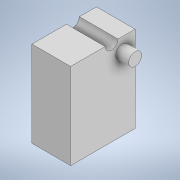
# Autodesk Inventor part: Support_1A
Saved by Autodesk Inventor 2021 (Build 250183000, 183)
## iProperties
Created: 2021-04-14
Part Number: Support_1A
Material: Generic
Document SubType Name: Modeling
Designer: Jawal
Density: 1 g/cm^3
Appearance: Default
Author: Jawal
Autodesk Inventor part; units mm, degrees
note: some values were not read from the file. Chosen so that the rebuilt part matches the saved one: direction of "Emboss1".
ref_plane "YZ Plane" through (0, 0, 0) normal (1, 0, 0) x (0, 1, 0)
ref_plane "XZ Plane" through (0, 0, 0) normal (0, 1, 0) x (-1, 0, 0)
ref_plane "XY Plane" through (0, 0, 0) normal (0, 0, 1) x (1, 0, 0)
sketch "Sketch1" plane through (0, 0, 0) normal (1, 0, 0) x (0, 1, 0)
  line L0 (10.5655, 7.5) -> (-10.5655, 7.5)
  line L1 (-10.5655, 7.5) -> (-10.5655, -6.983)
  line L2 (-10.5655, -6.983) -> (10.5655, -6.983)
  line L3 (10.5655, -6.983) -> (10.5655, 7.5)
  point P0 (0, 0)
  dimension "d0" = 21.131
  dimension "d2" = 10.5655
  dimension "d3" = 7.5
  dimension "d27" = 14.483
  constraints: 8 end point, 2 parallel, 1 horizontal, 1 perpendicular
  measures "d0" distance of L1.end L2.end
  measures "d2" distance from line of L3 point (0, 0)
  measures "d3" distance from line of L0 point (0, 0)
  measures "d27" distance of L0.start L2.end
extrude "Extrusion1" add sketch "Sketch1" along normal blind 9
sketch "Sketch3" plane through (9, 0, 0) normal (1, 0, 0) x (0, 0, -1)
  circle A0 centre (3.983, 6.2605) radius 1.5
  point P0 (0, 0)
  dimension "d12" = 3
  constraints: 1 centre point
  measures "d12" diameter of A0
extrude "Extrusion3" add sketch "Sketch3" along normal blind 3
sketch "Sketch4" plane through (0, 0, 0) normal (-1, 0, 0) x (0, 0, 1)
  line L0 (-2.5186, -3.6831) -> (10.3419, -3.6831) construction
  line L1 (10.3419, -3.6831) -> (10.3419, -8.8157) construction
  line L2 (10.3419, -8.8157) -> (-2.5186, -8.8157) construction
  line L3 (-2.5186, -8.8157) -> (-2.5186, -3.6831) construction
  line L4 (-0.5697, -6.741) -> (-2.0567, -6.741)
  line L5 (-2.0567, -6.741) -> (-2.0567, -6.4297)
  line L6 (-2.0567, -6.4297) -> (-1.5034, -6.4297)
  line L7 (-1.5034, -6.4297) -> (-1.5034, -4.387)
  line L8 (-1.5034, -4.387) -> (-2.0567, -4.387)
  line L9 (-2.0567, -4.387) -> (-2.0567, -4.1079)
  spline S0 degree 2 poles (-2.0567, -4.1079) (-1.743, -4.1079) (-1.4466, -3.9301) (-1.4268, -3.6831) knots 0 0 0 1 2 2 2
  line L10 (-1.4268, -3.6831) -> (-1.1106, -3.6831)
  line L11 (-1.1106, -3.6831) -> (-1.1106, -6.4297)
  line L12 (-1.1106, -6.4297) -> (-0.5697, -6.4297)
  line L13 (-0.5697, -6.4297) -> (-0.5697, -6.741)
  line L14 (-0.2511, -6.741) -> (0.7764, -3.693)
  line L15 (0.7764, -3.693) -> (1.2754, -3.693)
  line L16 (1.2754, -3.693) -> (2.3029, -6.741)
  line L17 (2.3029, -6.741) -> (1.8756, -6.741)
  line L18 (1.8756, -6.741) -> (1.599, -5.8888)
  line L19 (1.599, -5.8888) -> (0.4356, -5.8888)
  line L20 (0.4356, -5.8888) -> (0.1589, -6.741)
  line L21 (0.1589, -6.741) -> (-0.2511, -6.741)
  line L22 (1.4878, -5.543) -> (1.016, -4.1079)
  line L23 (1.016, -4.1079) -> (0.5467, -5.543)
  line L24 (0.5467, -5.543) -> (1.4878, -5.543)
  point P0 (0, 0)
  constraints: 2 other
emboss "Emboss1" sketch "Sketch4" operation cut depth 1 direction (1, 0, 0)
sketch "Sketch6" plane through (0, -10.5655, -6.983) normal (0, -1, 0) x (1, 0, 0)
  line L0 (0, 14.483) -> (0, 0) projected
  line L1 (9, 14.483) -> (9, 0) projected
  line L2 (0, 0) -> (9, 0)
  line L3 (9, 0) -> (9, 14.483)
  line L4 (9, 14.483) -> (0, 14.483)
  line L5 (0, 14.483) -> (0, 0)
  point P0 (0, 6.983)
  constraints: 8 end point, 2 parallel, 1 horizontal, 1 perpendicular
extrude "Extrusion5" add sketch "Sketch6" along normal blind 0.174
sketch "Sketch7" plane through (0, 10.5655, 7.5) normal (0, 0, 1) x (1, 0, 0)
  line L0 (0, 0) -> (9, 0) projected
  line L1 (9, 0) -> (9, -21.305) projected
  line L2 (0, 0) -> (9, 0)
  line L3 (9, 0) -> (9, -21.305)
  line L4 (9, -21.305) -> (0, -21.305)
  line L5 (0, -21.305) -> (0, 0)
  point P0 (0, -10.5655)
  constraints: 8 end point, 2 parallel, 1 horizontal, 1 perpendicular
extrude "Extrusion6" add sketch "Sketch7" along normal blind 0.517
sketch "Sketch10" plane through (0, 10.5655, 8.017) normal (0, 1, 0) x (1, 0, 0)
  line L0 (0, 15) -> (9, 15) projected
  line L1 (9, 15) -> (9, 0) projected
  line L2 (0, 15) -> (9, 15)
  line L3 (9, 15) -> (9, 0)
  line L4 (9, 0) -> (0, 0)
  line L5 (0, 0) -> (0, 15)
  point P0 (0, 8.017)
  point P1 (9, 8.019)
  point P2 (9, 8.019)
  constraints: 8 end point, 2 parallel, 1 horizontal, 1 perpendicular
extrude "Extrusion9" cut sketch "Sketch10" against normal blind 1.302
sketch "Sketch11" plane through (0, 0, 0) normal (-1, 0, 0) x (0, 0, 1)
  circle A0 centre (-1.502, 9.3028) radius 1.5
  line L0 (8.017, 9.2635) -> (8.017, -10.7395) projected
  point P0 (0, 0)
  dimension "d40" = 3
  dimension "d41" = 9.519
  constraints: 1 centre point
  measures "d40" diameter of A0
  measures "d41" distance from line of L0 A0.centre
extrude "Extrusion10" cut sketch "Sketch11" against normal up to surface (9 mm away)
equation "\"d2\" = 0.5 * d0"
body "Solid1"
